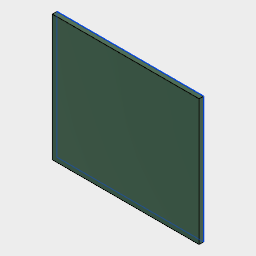
Board (Autodesk Fusion 360 design; units mm, degrees)
Autodesk Fusion 360 part; units mm, degrees
sketch "sketch 259" plane through (6.625, 39.38, 0) normal (0, 0, 1) x (1, 0, 0)
  line L0 (-6.625, -39.38) -> (43.375, -39.38)
  line L1 (43.375, 3.62) -> (43.375, -39.38)
  line L2 (-6.625, 3.62) -> (43.375, 3.62)
  line L3 (-6.625, -39.38) -> (-6.625, 3.62)
extrude "Extrude1" add sketch "sketch 259" along normal blind 1.57
named bodies: "Board"
